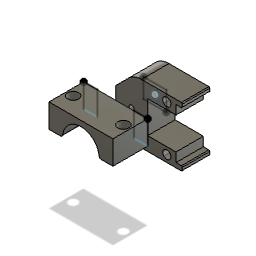
weatherstation_mounts (Autodesk Fusion 360 design; units mm, degrees)
Autodesk Fusion 360 part; units mm, degrees
sketch "Skizze1" plane through (0, 0, 0) normal (0, 1, 0) x (1, 0, 0)
  line L0 (0, 0) -> (70, 0)
  line L1 (70, 0) -> (70, -38)
  line L2 (70, -38) -> (0, -38)
  line L3 (0, -38) -> (0, 0)
  line L4 (0, 0) -> (15, 0)
  line L5 (15, 0) -> (15, -38)
  line L6 (15, -38) -> (0, -38)
  line L7 (0, -38) -> (0, 0)
  line L8 (70, 0) -> (55, 0)
  line L9 (55, 0) -> (55, -38)
  line L10 (55, -38) -> (70, -38)
  line L11 (70, -38) -> (70, 0)
  circle A0 centre (62.5, -19) radius 4.5
  circle A1 centre (7.5, -19) radius 4.5
  dimension "d1" = 70
  dimension "d2" = 38
  dimension "d3" = 15
  dimension "d4" = 15
  dimension "d5" = 9
  dimension "d6" = 9
  constraint horizontal L0
  constraint vertical L1
  constraint horizontal L2
  constraint vertical L3
  constraint coincident L0.start L3.end
  constraint horizontal L4
  constraint vertical L5
  constraint horizontal L6
  constraint vertical L7
  constraint horizontal L8
  constraint vertical L9
  constraint horizontal L10
  constraint vertical L11
  measures "d1" distance of L0.start L0.end
  measures "d2" distance of L0.start L2.end
  measures "d3" distance of L0.start L4.end
  measures "d4" distance of L0.end L8.end
  measures "d5" diameter of A0
  measures "d6" diameter of A1
extrude "Extrusion1" add sketch "Skizze1" along normal blind 26 makes body 1
sketch "Skizze2" plane through (0, 0, 0) normal (0, 0, -1) x (-1, 0, 0)
  line L0 (-70, 0) -> (0, 0)
  line L1 (0, 0) -> (0, 26)
  line L2 (0, 26) -> (-70, 26)
  line L3 (-70, 26) -> (-70, 0)
  line L4 (0, 0) -> (-15, 0)
  line L5 (-15, 0) -> (-15, 26)
  line L6 (-15, 26) -> (0, 26)
  line L7 (0, 26) -> (0, 0)
  line L8 (-70, 0) -> (-55, 0)
  line L9 (-55, 0) -> (-55, 26)
  line L10 (-55, 26) -> (-70, 26)
  line L11 (-70, 26) -> (-70, 0)
  circle A0 centre (-35, 0) radius 20
  dimension "d9" = 15
  dimension "d10" = 15
  constraint horizontal L4
  constraint vertical L5
  constraint horizontal L6
  constraint vertical L7
  constraint coincident L0.end L1.start
  constraint horizontal L8
  constraint vertical L9
  constraint horizontal L10
  constraint vertical L11
  constraint coincident L0.start L3.end
  constraint midpoint L0 A0.centre
  constraint coincident L8.end A0
  measures "d9" distance of L0.end L4.end
  measures "d10" distance of L0.start L8.end
extrude "Extrusion2" cut sketch "Skizze2" against normal blind 100 contours L0 A0 picked at (-29.4917, 5.7427) bodies 1
fillet "Abrundung1" radius 2.5 2 edges at (15, 0, 19) (55, 0, 19) on bodies 1
sketch "Skizze3" plane through (0, 0, 0) normal (0, 0, -1) x (-1, 0, 0)
  arc A0 (-57.3607, 0) -> (-54.8762, 2.2222) centre (-57.3607, 2.5) ccw
  arc A1 (-15.1238, 2.2222) -> (-54.8762, 2.2222) centre (-35, 0) ccw
  arc A2 (-15.1238, 2.2222) -> (-12.6393, 0) centre (-12.6393, 2.5) ccw
  line L0 (-12.6393, 0) -> (0, 0)
  line L1 (0, 0) -> (0, 26)
  line L2 (0, 26) -> (-70, 26)
  line L3 (-70, 26) -> (-70, 0)
  line L4 (-70, 0) -> (-57.3607, 0)
  line L5 (0, 26) -> (-15, 26)
  line L6 (-15, 26) -> (-15, 0)
  line L7 (-15, 0) -> (0, 0)
  line L8 (0, 0) -> (0, 26)
  line L9 (-70, 26) -> (-55, 26)
  line L10 (-55, 26) -> (-55, 0)
  line L11 (-55, 0) -> (-70, 0)
  line L12 (-70, 0) -> (-70, 26)
  dimension "d15" = 15
  dimension "d16" = 15
  constraint horizontal L5
  constraint vertical L6
  constraint horizontal L7
  constraint vertical L8
  constraint coincident L1.end L2.start
  constraint horizontal L9
  constraint vertical L10
  constraint horizontal L11
  constraint vertical L12
  constraint coincident L2.end L3.start
  measures "d15" distance of L1.end L5.end
  measures "d16" distance of L2.end L9.end
ref_plane "Arbeitsebene1" through (0, 0, -70) normal (0, 0, 1) x (1, 0, 0)
sketch "Skizze4" plane through (0, 0, -70) normal (0, 0, 1) x (1, 0, 0)
  line L0 (0, -75) -> (38, -75)
  line L1 (38, -75) -> (38, -60)
  line L2 (38, -60) -> (0, -60)
  line L3 (0, -60) -> (0, -75)
  line L4 (38, -67.5) -> (21, -67.5)
  circle A0 centre (21, -67.5) radius 4.5
  line L5 (38, -60) -> (31, -60)
  line L6 (31, -60) -> (31, -70)
  line L7 (31, -70) -> (38, -70)
  line L8 (38, -70) -> (38, -60)
  dimension "d18" = 38
  dimension "d19" = 15
  dimension "d20" = 17
  dimension "d21" = 9
  dimension "d22" = 7
  dimension "d23" = 10
  constraint horizontal L0
  constraint vertical L1
  constraint horizontal L2
  constraint vertical L3
  constraint midpoint L1 L4.start
  constraint perpendicular L1 L4
  constraint coincident L4.end A0.centre
  constraint horizontal L5
  constraint vertical L6
  constraint horizontal L7
  constraint vertical L8
  measures "d18" distance of L0.start L0.end
  measures "d19" distance of L0.start L2.end
  measures "d20" distance of L4.start L4.end
  measures "d21" diameter of A0
  measures "d22" distance of L1.end L5.end
  measures "d23" distance of L1.end L7.end
extrude "Extrusion3" add sketch "Skizze4" against normal blind 30 separate body contours L0 L1 L2 L3 L6 L7 makes body 2
copy_body "Körper kopieren/einfügen1" bodies 2 makes body 3
mirror "Spiegeln1" about plane through (0, 0, -100) normal (0, 0, 1) of bodies 2 makes body 4
move_body "Verschieben1" bodies 4 to x (1, 0, 0) y (0, 1, 0) z (0, 0, 1) at (0, 0, -35)
move_body "Verschieben2" bodies 4 to x (1, 0, 0) y (0, -1, 0) z (0, 0, -1) at (0, -85, -235)
sketch "Skizze5" plane through (0, 0, 0) normal (-1, 0, 0) x (0, 0, 1)
  line L0 (-70, -25) -> (-70, -10)
  line L1 (-70, -10) -> (-100, -10)
  line L2 (-100, -10) -> (-100, -25)
  line L3 (-100, -25) -> (-70, -25)
  line L4 (-100, -10) -> (-70, -10)
  line L5 (-70, -10) -> (-70, -75)
  line L6 (-70, -75) -> (-100, -75)
  line L7 (-100, -75) -> (-100, -10)
  constraint horizontal L4
  constraint vertical L5
  constraint horizontal L6
  constraint vertical L7
  constraint coincident L1.end L2.start
extrude "Extrusion4" add sketch "Skizze5" along normal blind 30 bodies 2 3 4
sketch "Skizze6" plane through (-30, 0, 0) normal (-1, 0, 0) x (0, 0, 1)
  line L0 (-100, -75) -> (-70, -75)
  line L1 (-70, -75) -> (-70, -10)
  line L2 (-70, -10) -> (-100, -10)
  line L3 (-100, -10) -> (-100, -75)
  line L4 (-100, -10) -> (-70, -10)
  line L5 (-70, -10) -> (-70, -75)
  line L6 (-70, -75) -> (-100, -75)
  line L7 (-100, -75) -> (-100, -10)
  line L8 (-74.5, -53) -> (-95.5, -53)
  line L9 (-95.5, -53) -> (-95.5, -32)
  line L10 (-95.5, -32) -> (-74.5, -32)
  line L11 (-74.5, -32) -> (-74.5, -53)
  line L12 (-74.5, -53) -> (-95.5, -32) construction
  line L13 (-95.5, -53) -> (-74.5, -32) construction
  point P0 (-85, -42.5)
  dimension "d30" = 21
  dimension "d31" = 21
  constraint horizontal L4
  constraint vertical L5
  constraint horizontal L6
  constraint vertical L7
  constraint coincident L0.end L1.start
  constraint coincident L2.end L3.start
  constraint horizontal L8
  constraint perpendicular L8 L9
  constraint parallel L8 L10
  constraint parallel L9 L11
  constraint coincident L12 P0
  constraint coincident L13 P0
  measures "d30" distance of L9.end L10.end
  measures "d31" distance of L8.end L9.end
extrude "Extrusion5" cut sketch "Skizze6" against normal blind 25 contours L8 L9 L10 L11 bodies 2
sketch "Skizze7" plane through (0, 0, -95.5) normal (0, 0, 1) x (1, 0, 0)
  line L0 (-30, -32) -> (-30, -53)
  line L1 (-30, -53) -> (-5, -53)
  line L2 (-5, -53) -> (-5, -32)
  line L3 (-5, -32) -> (-30, -32)
  line L4 (-5, -53) -> (-30, -53)
  line L5 (-30, -53) -> (-30, -32)
  line L6 (-30, -32) -> (-5, -32)
  line L7 (-5, -32) -> (-5, -53)
  circle A0 centre (-17.5, -42.5) radius 2.75
  dimension "d34" = 5.5
  constraint horizontal L4
  constraint vertical L5
  constraint horizontal L6
  constraint vertical L7
  constraint coincident L0.start L3.end
  constraint coincident L1.end L2.start
  measures "d34" diameter of A0
extrude "Extrusion6" cut sketch "Skizze7" along normal blind 37 contours A0 bodies 2
extrude "Extrusion7" cut sketch "Skizze7" against normal blind 10 contours A0 bodies 2
extrude "Extrusion8" add 1 faces at (-30, -67.6667, -81.5) along direction (-1, 0, 0) blind 5 on bodies 2 bodies 2
chamfer "Fase1" distance 20 angle 45 2 edges at (-35, -75, -85) (-35, -10, -85) on bodies 2
fillet "Abrundung2" radius 1 4 edges at (38, -15, -85) (38, -10, -85) (38, -75, -85) (38, -70, -85) on bodies 2
fillet "Abrundung3" radius 20 2 edges at (-15, -75, -85) (-15, -10, -85) on bodies 2
sketch "Skizze8" plane through (0, 26, 0) normal (0, 1, 0) x (-1, 0, 0)
  circle A0 centre (-7.5, 19) radius 4.5
  circle A1 centre (-62.5, 19) radius 4.5
  line L0 (0, 38) -> (-70, 38)
  line L1 (-70, 38) -> (-70, 0)
  line L2 (-70, 0) -> (0, 0)
  line L3 (0, 0) -> (0, 38)
  circle A2 centre (-7.5, 19) radius 6
  circle A3 centre (-62.5, 19) radius 6
  dimension "d46" = 12
  dimension "d47" = 12
  constraint concentric A0 A2
  constraint concentric A1 A3
  measures "d46" diameter of A2
  measures "d47" diameter of A3
extrude "Extrusion9" cut sketch "Skizze8" against normal blind 20 contours A2 | A3 bodies 1
